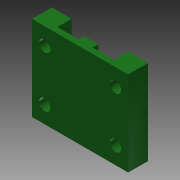
# Autodesk Inventor part: Linear Bearing Platform Adapter Back
Saved by Autodesk Inventor 2015 SP1 (Build 190203100, 203)
## iProperties
Created: 2015-03-04
Part Number: Linear Bearing Platform Adapter Back
Material: PC/ABS Plastic
Document SubType Name: Modeling
Designer: Andrew
Density: 0.357273 g/cm^3
Appearance: Smooth - Dark Forest Green
Author: Andrew
Autodesk Inventor part; units mm, degrees
ref_plane "YZ Plane" through (0, 0, 0) normal (1, 0, 0) x (0, 1, 0)
ref_plane "XZ Plane" through (0, 0, 0) normal (0, 1, 0) x (-1, 0, 0)
ref_plane "XY Plane" through (0, 0, 0) normal (0, 0, 1) x (1, 0, 0)
sketch "Sketch1" plane through (0, 0, 0) normal (0, 1, 0) x (-1, 0, 0)
  line L0 (-17, 15) -> (17, 15)
  line L1 (17, 15) -> (17, -15)
  line L2 (17, -15) -> (-17, -15)
  line L3 (-17, -15) -> (-17, 15)
  line L4 (-17, 15) -> (17, -15) construction
  line L5 (17, 15) -> (-17, -15) construction
  line L6 (-10, 15) -> (10, 15)
  line L7 (10, 15) -> (10, -15)
  line L8 (10, -15) -> (-10, -15)
  line L9 (-10, -15) -> (-10, 15)
  line L10 (-10, 15) -> (10, -15) construction
  line L11 (10, 15) -> (-10, -15) construction
  line L12 (-2.5, 15) -> (2.5, 15)
  line L13 (2.5, 15) -> (2.5, -15)
  line L14 (2.5, -15) -> (-2.5, -15)
  line L15 (-2.5, -15) -> (-2.5, 15)
  line L16 (-2.5, 15) -> (2.5, -15) construction
  line L17 (2.5, 15) -> (-2.5, -15) construction
  point P0 (0, 0)
  point P1 (12.5, 9)
  dimension "d0" = 20
  dimension "d1" = 5
  dimension "d2" = 34
  dimension "d3" = 30
  dimension "d4" = 6
  dimension "d5" = 4.5
  constraints: 36 end point, 6 midpoint, 6 parallel, 3 horizontal, 3 perpendicular, 2 point on line
  measures "d0" distance between parallel lines of L9 L7
  measures "d1" distance between parallel lines of L15 L13
  measures "d2" distance of L1.end L2.end
  measures "d3" distance of L2.end L0.start
  measures "d4" distance from line of L0 point (12.5, 9)
  measures "d5" distance from line of L1 point (12.5, 9)
extrude "Extrusion1" add sketch "Sketch1" along normal blind 2 contours L0 L15 L2 L9 | L0 L7 L2 L13
extrude "Extrusion2" add sketch "Sketch1" along normal blind 7 contours L0 L9 L2 L3 | L0 L1 L2 L7
extrude "Extrusion3" add sketch "Sketch1" along normal blind 4 contours L0 L13 L2 L15
hole "Hole1" at (-12.5, 0, 9) direction (0, 1, 0) diameter 4 end through all
pattern_linear "Rectangular Pattern1" count 2 spacing 18 along (0, 0, -1) count 2 spacing 25 along (1, 0, 0) of "Hole1"
body "Solid1"
